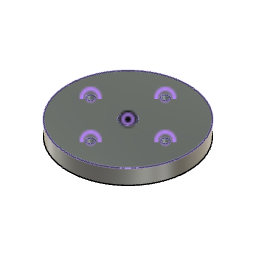
circletopcap v1 (Autodesk Fusion 360 design; units mm, degrees)
Autodesk Fusion 360 part; units mm, degrees
sketch "Sketch1" plane through (0, 0, 0) normal (0, 0, 1) x (1, 0, 0)
  circle A0 centre (0, 0) radius 50.8
  line L0 (0, 0) -> (0, 31.75) construction
  circle A1 centre (0, 31.75) radius 3
  circle A2 centre (-31.75, 0) radius 3
  circle A3 centre (0, -31.75) radius 3
  circle A4 centre (31.75, 0) radius 3
  circle A5 centre (0, 0) radius 6
  dimension "d1" = 101.6
  dimension "d2" = 31.75
  dimension "d3" = 6
  dimension "d5" = 360
  dimension "d6" = 12
  constraint coincident A0.centre L0.start
  constraint vertical L0
  constraint coincident L0.end A1.centre
  measures "d1" diameter of A0
  measures "d2" distance of A0.centre L0.end
  measures "d3" diameter of A1
  measures "d6" diameter of A5
extrude "Extrude1" add sketch "Sketch1" along normal blind 12.7
sketch "Sketch2" plane through (0, 0, 12.7) normal (0, 0, 1) x (-1, 0, 0)
  circle A0 centre (0, -31.75) radius 3
  circle A1 centre (31.75, 0) radius 3
  circle A2 centre (0, 31.75) radius 3
  circle A3 centre (-31.75, 0) radius 3
  circle A4 centre (0, 0) radius 6
  circle A5 centre (0, 0) radius 50.8
equation "d2 = 2.5 in / 2"
